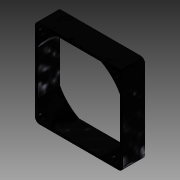
# Autodesk Inventor part: 60mm Fan Footprint
Saved by Autodesk Inventor 2015 (Build 190159000, 159)
## iProperties
Created: 2015-05-12
Part Number: 60mm Fan Footprint
Material: ABS Plastic
Document SubType Name: Modeling
Designer: carpenma
Density: 1.06 g/cm^3
Appearance: Black
Author: carpenma
Autodesk Inventor part; units mm, degrees
ref_plane "YZ Plane" through (0, 0, 0) normal (1, 0, 0) x (0, 1, 0)
ref_plane "XZ Plane" through (0, 0, 0) normal (0, 1, 0) x (-1, 0, 0)
ref_plane "XY Plane" through (0, 0, 0) normal (0, 0, 1) x (1, 0, 0)
sketch "Sketch1" plane through (0, 0, 0) normal (0, 0, 1) x (1, 0, 0)
  line L0 (0, 0) -> (60, 0)
  line L1 (60, 0) -> (60, -60)
  line L2 (60, -60) -> (0, -60)
  line L3 (0, -60) -> (0, 0)
  dimension "d0" = 60
  dimension "d1" = 60
  constraints: 8 end point, 2 parallel, 1 horizontal, 1 perpendicular
  measures "d0" distance of L1.end L2.end
  measures "d1" distance of L0.end L1.end
extrude "Extrusion1" add sketch "Sketch1" against normal blind 15
sketch "Sketch2" plane through (0, 0, 0) normal (0, 0, 1) x (1, 0, 0)
  line L0 (0, 0) -> (60, 0) projected
  line L1 (0, -60) -> (0, 0) projected
  line L2 (60, -60) -> (0, -60) projected
  line L3 (60, 0) -> (60, -60) projected
  circle A0 centre (5, -5) radius 2.15
  circle A1 centre (55, -5) radius 2.15
  circle A2 centre (55, -55) radius 2.15
  circle A3 centre (5, -55) radius 2.15
  dimension "d5" = 4.3
  dimension "d6" = 4.3
  dimension "d7" = 4.3
  dimension "d8" = 4.3
  dimension "d9" = 50
  dimension "d10" = 50
  dimension "d11" = 5
  dimension "d12" = 5
  constraints: 4 centre point, 2 horizontal alignment, 2 vertical alignment
  measures "d5" diameter of A0
  measures "d6" diameter of A1
  measures "d7" diameter of A3
  measures "d8" diameter of A2
  measures "d9" distance of A1.centre A0.centre
  measures "d10" distance of A0.centre A3.centre
  measures "d11" distance from line of L1 A0.centre
  measures "d12" distance from line of L0 A0.centre
extrude "Extrusion2" cut sketch "Sketch2" against normal up to next contours A0 | A1 | A2 | A3
sketch "Sketch3" plane through (0, 0, 0) normal (0, 0, 1) x (1, 0, 0)
  circle A0 centre (55, -55) radius 2.15 projected
  circle A1 centre (5, -5) radius 2.15 projected
  circle A2 centre (55, -5) radius 2.15 projected
  circle A3 centre (5, -55) radius 2.15 projected
  line L0 (0, 0) -> (60, 0) projected
  line L1 (0, -60) -> (0, 0) projected
  line L2 (60, -60) -> (0, -60) projected
  line L3 (60, 0) -> (60, -60) projected
  line L4 (15.0313, -2) -> (44.9687, -2)
  line L5 (2, -44.9687) -> (2, -15.0313)
  line L6 (44.9687, -58) -> (15.0313, -58)
  line L7 (58, -15.0313) -> (58, -44.9687)
  arc A4 (15.0313, -2) -> (2, -15.0313) centre (30, -30) ccw
  arc A5 (2, -44.9687) -> (15.0313, -58) centre (30, -30) ccw
  arc A6 (44.9687, -58) -> (58, -44.9687) centre (30, -30) ccw
  arc A7 (58, -15.0313) -> (44.9687, -2) centre (30, -30) ccw
  dimension "d23" = 360
  dimension "d16" = 60
  dimension "d17" = 30
  dimension "d18" = 30
  dimension "d20" = 2
  constraints: 8 end point, 8 point on circle, 4 centre point, 1 horizontal, 13 other
  measures "d16" distance of L0.start L0.end
  measures "d17" distance from line of L1 A4.centre
  measures "d18" distance from line of L0 A4.centre
  measures "d20" distance between parallel lines of L0 L4
extrude "Extrusion3" cut sketch "Sketch3" against normal up to next contours L4 A7 L7 A6 L6 A5 L5 A4
fillet "Fillet2" radius 3.175 4 edges at (0, 0, -7.5) (0, -60, -7.5) (60, -60, -7.5) (60, 0, -7.5)
equation "\"d1\" = d0"
equation "\"d6\" = d5"
equation "\"d7\" = d5"
equation "\"d8\" = d5"
equation "\"d10\" = d9"
equation "\"d12\" = d11"
equation "\"d17\" = 0.5 * d16"
equation "\"d18\" = d17"
body "Solid1"
